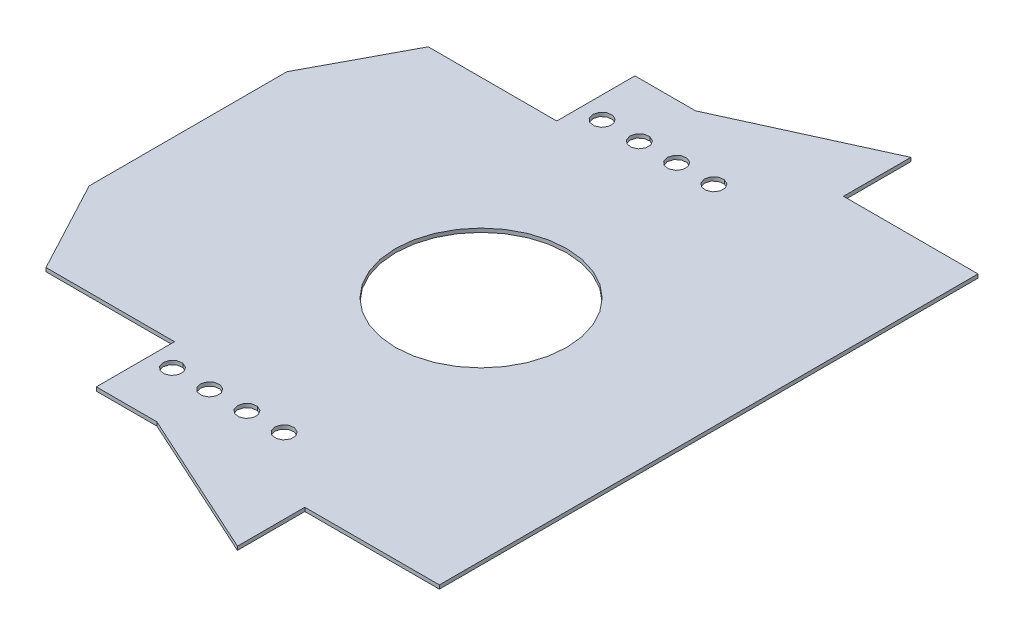
# Autodesk Inventor part: base_1
Saved by Autodesk Inventor 2023 (Build 270158000, 158)
## iProperties
Created: 2023-08-10
Part Number: base_1
Material: Genérico
Document SubType Name: Modeling
Designer: azeve
Density: 1 g/cm^3
Appearance: Padrão
Author: azeve
Autodesk Inventor part; units mm, degrees
ref_plane "YZ Plane" through (0, 0, 0) normal (1, 0, 0) x (0, 1, 0)
ref_plane "XZ Plane" through (0, 0, 0) normal (0, 1, 0) x (-1, 0, 0)
ref_plane "XY Plane" through (0, 0, 0) normal (0, 0, 1) x (1, 0, 0)
sketch "Esboço1" plane through (0, 0, 0) normal (0, 1, 0) x (-1, 0, 0)
  line L0 (139.8134, -26.55) -> (126.6305, -51.3208)
  line L1 (139.8134, -26.55) -> (139.8134, 0)
  line L2 (139.8134, -26.55) -> (126.6305, -51.3208)
  circle A0 centre (61.129, 0) radius 23
  circle A1 centre (56.3183, -57.6959) radius 2.5
  circle A2 centre (76.3183, -57.6959) radius 2.5
  circle A3 centre (86.3183, -57.6959) radius 2.5
  circle A4 centre (66.3183, -57.6959) radius 2.5
  line L3 (92.1195, -55.1192) -> (92.1195, -72.3197)
  line L4 (75.8622, -72.3197) -> (92.1195, -72.3197)
  line L5 (36.1237, -90.4148) -> (36.1237, -72.3197)
  line L6 (75.8622, -72.3197) -> (36.1237, -90.4148)
  line L7 (126.6305, -51.3208) -> (92.1195, -51.3208)
  line L8 (92.1195, -51.3208) -> (92.1195, -55.1192)
  line L9 (139.8134, 26.55) -> (126.6305, 51.3208)
  line L10 (139.8134, 26.55) -> (139.8134, 0)
  circle A5 centre (76.3183, 57.6959) radius 2.5
  circle A6 centre (86.3183, 57.6959) radius 2.5
  circle A7 centre (66.3183, 57.6959) radius 2.5
  circle A8 centre (56.3183, 57.6959) radius 2.5
  line L11 (92.1195, 55.1192) -> (92.1195, 72.3197)
  line L12 (75.8622, 72.3197) -> (92.1195, 72.3197)
  line L13 (36.1237, 90.4148) -> (36.1237, 72.3197)
  line L14 (75.8622, 72.3197) -> (36.1237, 90.4148)
  line L15 (126.6305, 51.3208) -> (92.1195, 51.3208)
  line L16 (92.1195, 51.3208) -> (92.1195, 55.1192)
  line L17 (0, 65.2411) -> (0, -65.2411)
  line L18 (36.1237, 72.3197) -> (0, 72.3197)
  line L19 (0, 72.3197) -> (0, 65.2411)
  line L20 (36.1237, -72.3197) -> (0, -72.3197)
  line L21 (0, -72.3197) -> (0, -65.2411)
  point P0 (0, 0)
  dimension "d1" = 46
  dimension "d6" = 130.4821
  constraints: 44 end point, 9 centre point, 4 perpendicular, 4 vertical, 2 horizontal, 2 point on line, 1 collinear
  measures "d1" diameter of A0
  measures "d6" distance of L17.start L17.end
extrude "Extrusão1" add sketch "Esboço1" along normal blind 1
